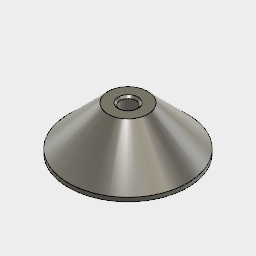
wedge (Autodesk Fusion 360 design; units mm, degrees)
Autodesk Fusion 360 part; units mm, degrees
sketch "Sketch1" plane through (0, 0, 0) normal (0, 1, 0) x (1, 0, 0)
  circle A0 centre (0, 0) radius 30
  circle A1 centre (0, 0) radius 4
  dimension "d1" = 60
  dimension "d3" = 8
  measures "d1" diameter of A0
  measures "d3" diameter of A1
extrude "Extrude1" add sketch "Sketch1" along normal blind 60
chamfer "Chamfer1" distance 20 angle 45 1 edges at (-27.9698, 60, 10.8485) measured on face at (21.2216, 60, 1.4904)
sketch "Sketch2" plane through (0, 0, 0) normal (0, 1, 0) x (1, 0, 0)
  circle A0 centre (0, 0) radius 11
  dimension "d8" = 22
  measures "d8" diameter of A0
extrude "Extrude2" cut sketch "Sketch2" along normal blind 8
extrude "Extrude3" cut 1 faces at (23.514, 0, 2.0369) along direction (0, 1, 0) blind 38
extrude "Extrude4" cut 1 faces at (8.6257, 8, 0.5465) along direction (0, 1, 0) blind 38
extrude "Extrude5" add 1 faces at (8.6257, 46, 0.5465) along direction (0, -1, 0) blind 0.5
chamfer "Chamfer2" distance 7 angle 45 1 edges at (-3.7293, 45.5, 1.4465) measured on face at (8.6257, 45.5, 0.5465)
chamfer "Chamfer3" distance 2 angle 45 1 edges at (-10.2556, 38, -3.9778) measured on face at (10.9453, 43, 1.0952)
chamfer "Chamfer4" distance 1 angle 45 1 edges at (-3.7293, 60, -1.4465) measured on face at (7.9479, 60, 0.6955)
